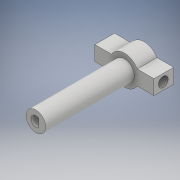
# Autodesk Inventor part: Stepper_Key
Saved by Autodesk Inventor 2017 (Build 210142000, 142)
## iProperties
Created: 2017-03-17
Part Number: Stepper_Key
Material: Generic
Document SubType Name: Modeling
Designer: s4321966
Density: 1 g/cm^3
Appearance: Default
Author: s4321966
Autodesk Inventor part; units mm, degrees
ref_plane "YZ Plane" through (0, 0, 0) normal (1, 0, 0) x (0, 1, 0)
ref_plane "XZ Plane" through (0, 0, 0) normal (0, 1, 0) x (-1, 0, 0)
ref_plane "XY Plane" through (0, 0, 0) normal (0, 0, 1) x (1, 0, 0)
sketch "Sketch3" plane through (0, 0, 0) normal (0, 1, 0) x (-1, 0, 0)
  circle A0 centre (0, 0) radius 7.5
  line L0 (0, 0) -> (15, 0)
  line L1 (0, 0) -> (15, 0) construction
  line L2 (15, 0) -> (15, -3.75)
  line L3 (15, -3.75) -> (-15, -3.75)
  line L4 (-15, -3.75) -> (-15, 3.75)
  line L5 (-15, 3.75) -> (15, 3.75)
  line L6 (15, 3.75) -> (15, -3.75)
  dimension "d27" = 15
  dimension "d28" = 15
  dimension "d29" = 0
  dimension "d30" = 3.75
  dimension "d31" = 90
  dimension "d32" = 30
  dimension "d33" = 7.5
  constraints: 14 end point, 3 horizontal, 2 parallel, 2 perpendicular, 1 centre point, 1 coincident, 1 collinear
  measures "d27" diameter of A0
  measures "d28" distance of L0.start L0.end
  measures "d29" distance between parallel lines of L0 L1
  measures "d30" distance of L0.end L2.end
  measures "d31" angle of L0 L2
  measures "d32" distance of L4.end L5.end
  measures "d33" distance of L3.end L4.end
extrude "Extrusion3" add sketch "Sketch3" along normal blind 10
sketch "Sketch5" plane through (0, 0, 0) normal (0, -1, 0) x (1, 0, 0)
  circle A0 centre (0, 0) radius 5
  line L0 (0, 2.5) -> (0, -2.5) projected
  dimension "d39" = 10
  constraints: 1 centre point, 1 coincident
  measures "d39" diameter of A0
extrude "Extrusion5" add sketch "Sketch5" along normal blind 45
sketch "Sketch6" plane through (0, 10, 0) normal (0, 1, 0) x (1, 0, 0)
  circle A0 centre (0, 0) radius 2.5
  dimension "d44" = 5
  constraints: 1 centre point, 1 coincident
  measures "d44" diameter of A0
extrude "Extrusion6" cut sketch "Sketch6" against normal blind 60
sketch "Sketch7" plane through (0, 10, 0) normal (0, 1, 0) x (1, 0, 0)
  line L0 (0, 0) -> (2.5, 0)
  line L1 (2.5, 0) -> (1.5, 0)
  line L2 (2.5, 0) -> (3.5, 0) construction
  line L3 (1.5, 0) -> (1.5, -3.2812)
  line L4 (1.5, -3.2812) -> (1.5, 3.3122)
  arc A0 (1.5, -2) -> (1.5, 2) centre (0, 0) ccw
  line L5 (1.5, -2) -> (1.5, 2)
  dimension "d50" = 1
  dimension "d51" = 180
  constraints: 12 end point, 3 point on circle, 2 collinear, 2 horizontal, 2 point on line, 2 vertical, 1 centre point, 1 coincident
  measures "d50" distance of L0.end L1.end
  measures "d51" angle of L1 L2
extrude "Extrusion9" add sketch "Sketch7" against normal blind 55
sketch "Sketch8" plane through (15, 0, 3.75) normal (1, 0, 0) x (0, 0, -1)
  line L0 (0, 0) -> (0, 10) projected
  line L1 (0, 0) -> (7.5, 0) projected
  circle A0 centre (3.75, 4.7055) radius 2.5
  point P0 (3.75, 0)
  dimension "d58" = 5
  constraints: 1 centre point
  measures "d58" diameter of A0
extrude "Extrusion10" cut sketch "Sketch8" against normal blind 15
thread "Thread2" size "M5x0.8" class "6H" standard "ANSI Metric M Profile" full length
body "Solid3"
